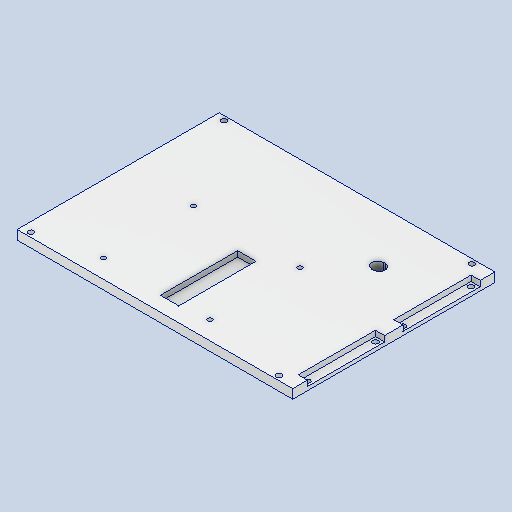
# Autodesk Inventor part: Camera plate
Saved by Autodesk Inventor 2023 (Build 270158000, 158)
## iProperties
Created: 2023-04-08
Part Number: Camera plate
Material: Aluminum 6061
Document SubType Name: Modeling
Designer: ASARe-DAQ-PC
Density: 2.7 g/cm^3
Appearance: Aluminum - Flat
Mass: 214.642 g
Surface Area: 362.73 cm^2
Volume: 79.497 cm^3
Author: ASARe-DAQ-PC
Autodesk Inventor part; units mm, degrees
ref_plane "YZ Plane" through (0, 0, 0) normal (1, 0, 0) x (0, 1, 0)
ref_plane "XZ Plane" through (0, 0, 0) normal (0, 1, 0) x (-1, 0, 0)
ref_plane "XY Plane" through (0, 0, 0) normal (0, 0, 1) x (1, 0, 0)
sketch "Sketch1" plane through (0, 0, 0) normal (0, 1, 0) x (-1, 0, 0)
  line L0 (0, 0) -> (150, 0)
  line L1 (150, 0) -> (150, -110)
  line L2 (150, -110) -> (0, -110)
  line L3 (0, -110) -> (0, 0)
  line L4 (40, -60) -> (0, -60)
  line L5 (0, -60) -> (0, -102)
  line L6 (0, -102) -> (40, -102)
  line L7 (40, -102) -> (40, -60)
  circle A0 centre (2.5, -62.5) radius 1.5
  circle A1 centre (2.5, -99.5) radius 1.5
  circle A2 centre (34.825, -81) radius 3.175
  circle A3 centre (33.825, -81) radius 3.175
  line L8 (34.825, -77.825) -> (33.825, -77.825)
  line L9 (34.825, -84.175) -> (33.825, -84.175)
  line L10 (37, -77.825) -> (37, -84.175) construction
  line L11 (25, -96) -> (0, -96)
  line L12 (0, -96) -> (0, -66)
  line L13 (0, -66) -> (25, -66)
  line L14 (25, -66) -> (25, -96)
  line L15 (5, -102) -> (5, -96)
  line L16 (5, -66) -> (5, -60)
  line L17 (5, -50) -> (0, -50)
  line L18 (0, -50) -> (0, -8)
  line L19 (0, -8) -> (5, -8)
  line L20 (5, -8) -> (5, -50)
  line L21 (5, -96) -> (5, -66)
  line L22 (80, -50) -> (70, -50)
  line L23 (70, -50) -> (70, -8)
  line L24 (70, -8) -> (80, -8)
  line L25 (80, -8) -> (80, -50)
  point P0 (0, -81)
  point P1 (40, -81)
  point P2 (0, -60)
  point P3 (25, -81)
  point P4 (5, -99)
  point P5 (0, -66)
  point P6 (0, -96)
  point P7 (0, -50)
  point P8 (70, -29)
  point P9 (5, -29)
  dimension "d0" = 110
  dimension "d3" = 42
  dimension "d6" = 40
  dimension "d13" = 3
  dimension "d14" = 3
  dimension "d18" = 2.5
  dimension "d19" = 2.5
  dimension "d20" = 2.5
  dimension "d21" = 2.5
  dimension "d22" = 6.35
  dimension "d23" = 1
  dimension "d26" = 37
  dimension "d29" = 25
  dimension "d30" = 30
  dimension "d31" = 5
  dimension "d32" = 150
  dimension "d33" = 8
  dimension "d34" = 42
  dimension "d35" = 5
  dimension "d36" = 8
  dimension "d73" = 10
  dimension "d74" = 42
  dimension "d75" = 70
  constraints: 52 end point, 12 point on line, 10 parallel, 7 horizontal, 7 perpendicular, 5 midpoint, 5 tangent, 4 centre point, 4 horizontal alignment, 4 point on circle, 1 collinear
  measures "d0" distance of L0.end L1.end
  measures "d3" distance of L6.end L4.start
  measures "d6" distance of L5.end L6.end
  measures "d13" diameter of A0
  measures "d14" diameter of A1
  measures "d18" distance from line of L4 A0.centre
  measures "d19" distance from line of L5 A0.centre
  measures "d20" distance from line of L3 A1.centre
  measures "d21" distance from line of L6 A1.centre
  measures "d22" diameter of A3
  measures "d23" distance of L9.start L9.end
  measures "d26" distance between parallel lines of L3 L10
  measures "d29" distance of L12.end L13.end
  measures "d30" distance of L13.end L11.start
  measures "d31" distance from line of L3 point (5, -99)
  measures "d32" distance of L0.start L0.end
  measures "d33" distance between parallel lines of L2 L6
  measures "d34" distance of L19.end L17.start
  measures "d35" distance of L18.end L19.end
  measures "d36" distance between parallel lines of L0 L19
  measures "d73" distance of L23.end L24.end
  measures "d74" distance of L22.end L23.end
  measures "d75" distance between parallel lines of L3 L23
extrude "Extrusion1" add sketch "Sketch1" against normal blind 5 contours L0 L1 L2 L3 L6 L7 L4 L17 L20 L19 | L19 L20 L17 L3 | L4 L16 L13 L3 | L3 L11 L15 L6 | L13 L21 L11 L3 | L4 L7 L6 L15 L11 L14 L13 L16 | L13 L14 L11 L21 | A0 | A1 | A2 A3 | A2 A3 L8 | L9 A3 A2 | A3 A2 | A2 A3 | L22 L23 L24 L25
extrude "Extrusion2" cut sketch "Sketch1" against normal blind 5 contours A0 | A1 | A2 A3 | A2 A3 L8 | L9 A3 A2 | A3 A2 | A2 A3
extrude "Extrusion3" cut sketch "Sketch1" against normal blind 3 contours L19 L20 L17 L3 | L4 L16 L13 L3 | L3 L11 L15 L6 | L13 L21 L11 L3 | L22 L23 L24 L25
sketch "Sketch2" plane through (0, -3, 0) normal (0, 1, 0) x (1, 0, 0)
  line L0 (-5, 50) -> (0, 50) projected
  line L1 (0, 50) -> (0, 8) projected
  line L2 (0, 8) -> (-5, 8) projected
  point P0 (0, 0)
  point P1 (-2.5, 47.5)
  point P2 (-2.5, 10.5)
  dimension "d44" = 2.5
  dimension "d45" = 2.5
  dimension "d46" = 2.5
  dimension "d47" = 2.5
  measures "d44" distance from line of L0 point (-2.5, 47.5)
  measures "d45" distance from line of L1 point (-2.5, 47.5)
  measures "d46" distance from line of L1 point (-2.5, 10.5)
  measures "d47" distance from line of L2 point (-2.5, 10.5)
hole "Hole1" at (-2.5, -3, -47.5) at (-2.5, -3, -10.5) direction (0, -1, 0) diameter 3 end through all
sketch "Sketch3" plane through (0, 0, 0) normal (0, 1, 0) x (1, 0, 0)
  line L0 (0, 0) -> (0, 8) projected
  line L1 (-150, 0) -> (0, 0) projected
  line L2 (0, 110) -> (-150, 110) projected
  line L3 (0, 102) -> (0, 110) projected
  point P0 (-10, 2.5)
  point P1 (-10, 107.5)
  dimension "d55" = 10
  dimension "d56" = 2.5
  dimension "d57" = 2.5
  dimension "d58" = 10
  measures "d55" distance from line of L0 point (-10, 2.5)
  measures "d56" distance from line of L1 point (-10, 2.5)
  measures "d57" distance from line of L2 point (-10, 107.5)
  measures "d58" distance from line of L3 point (-10, 107.5)
hole "Hole2" at (-10, 0, -2.5) at (-10, 0, -107.5) direction (0, -1, 0) diameter 3 depth 6 tip angle 118
pattern_linear "Rectangular Pattern1" count 2 spacing 135 along (-1, 0, 0) of "Hole2"
sketch "Sketch4" plane through (0, -5, 0) normal (0, -1, 0) x (1, 0, 0)
  line L0 (-113, -10) -> (-55, -10) construction
  line L1 (-55, -10) -> (-55, -59) construction
  line L2 (-55, -59) -> (-113, -59) construction
  line L3 (-113, -59) -> (-113, -10) construction
  line L4 (0, 0) -> (-150, 0) construction
  line L5 (0, -110) -> (0, 0) construction
  dimension "d69" = 58
  dimension "d70" = 49
  dimension "d71" = 10
  dimension "d72" = 55
  constraints: 8 end point, 3 coincident, 3 perpendicular, 1 horizontal
  measures "d69" distance of L0.start L0.end
  measures "d70" distance of L0.end L1.end
  measures "d71" distance from line of L4 L0.end
  measures "d72" distance between parallel lines of L1 L5
hole "Hole3" at (-113, -5, -10) at (-55, -5, -10) at (-55, -5, -59) at (-113, -5, -59) direction (0, 1, 0) diameter 2.459 end through all thread size "M3x0.5" class "6H" standard "ISO Metric profile"
body "Solid1"
